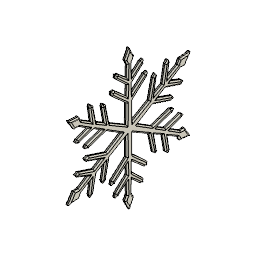
SnowFlake (Autodesk Fusion 360 design; units mm, degrees)
part number: 2026-06-10-18-37-35-509
Autodesk Fusion 360 part; units mm, degrees
sketch "Sketch1" plane through (0, 0, 0) normal (1, 0, 0) x (0, 1, 0)
  line L0 (-5.5093, 0.4362) -> (-18.2005, -7.4756)
  line L1 (-18.2005, -7.4756) -> (-32.6565, -2.7689)
  line L2 (-32.6565, -2.7689) -> (-35.5141, -3.6935)
  line L3 (-35.5141, -3.6935) -> (-34.2955, -5.7106)
  line L4 (-34.2955, -5.7106) -> (-22, -10)
  line L5 (-22, -10) -> (-28.4, -14)
  line L6 (-28.4, -14) -> (-40.4994, -10)
  line L7 (-40.4994, -10) -> (-42.867, -11.2872)
  line L8 (-42.867, -11.2872) -> (-41.5321, -12.9244)
  line L9 (-41.5321, -12.9244) -> (-32.5, -16.5)
  line L10 (-32.5, -16.5) -> (-40.363, -21.503)
  line L11 (-40.363, -21.503) -> (-44, -21.503)
  line L12 (-44, -21.503) -> (-48.7199, -28.8845)
  line L13 (-48.7199, -28.8845) -> (-40.1679, -28.1366)
  line L14 (-40.1679, -28.1366) -> (-38.477, -24.8523)
  line L15 (-38.477, -24.8523) -> (-30.5752, -19.9422)
  line L16 (-30.5752, -19.9422) -> (-32, -30)
  line L17 (-32, -30) -> (-31.2876, -32.0639)
  line L18 (-31.2876, -32.0639) -> (-28.76, -30)
  line L19 (-28.76, -30) -> (-26.2945, -17.4786)
  line L20 (-26.2945, -17.4786) -> (-19.6702, -13.6466)
  line L21 (-19.6702, -13.6466) -> (-21.809, -25.4099)
  line L22 (-21.809, -25.4099) -> (-21.0366, -27.3705)
  line L23 (-21.0366, -27.3705) -> (-18.779, -25.707)
  line L24 (-18.779, -25.707) -> (-15.8085, -11.5376)
  line L25 (-15.8085, -11.5376) -> (-2.5006, -3.7251)
  line L26 (-2.5006, -3.7251) -> (-2.2468, -18.655)
  line L27 (-2.2468, -18.655) -> (-14.0686, -29.3557)
  line L28 (-14.0686, -29.3557) -> (-14.5366, -32.1245)
  line L29 (-14.5366, -32.1245) -> (-11.9615, -32.0807)
  line L30 (-11.9615, -32.0807) -> (-2.2133, -23.506)
  line L31 (-2.2133, -23.506) -> (-1.8623, -31.1496)
  line L32 (-1.8623, -31.1496) -> (-10.9878, -39.6121)
  line L33 (-10.9878, -39.6121) -> (-11.3193, -42.4278)
  line L34 (-11.3193, -42.4278) -> (-9, -42)
  line L35 (-9, -42) -> (-2, -36)
  line L36 (-2, -36) -> (-1.7726, -45.2005)
  line L37 (-1.7726, -45.2005) -> (-3.5977, -48.4646)
  line L38 (-3.5977, -48.4646) -> (0.0525, -55.765)
  line L39 (0.0525, -55.765) -> (3.5974, -48.6752)
  line L40 (3.5974, -48.6752) -> (1.825, -45.1303)
  line L41 (1.825, -45.1303) -> (1.9829, -35.8293)
  line L42 (1.9829, -35.8293) -> (9, -42)
  line L43 (9, -42) -> (11.1435, -42.4628)
  line L44 (11.1435, -42.4628) -> (11.1906, -39.6913)
  line L45 (11.1906, -39.6913) -> (2, -31)
  line L46 (2, -31) -> (2.1281, -23.4568)
  line L47 (2.1281, -23.4568) -> (11.835, -31.9103)
  line L48 (11.835, -31.9103) -> (14.5094, -32.2339)
  line L49 (14.5094, -32.2339) -> (14.1643, -29.4085)
  line L50 (14.1643, -29.4085) -> (2.3645, -18.7108)
  line L51 (2.3645, -18.7108) -> (2.5306, -3.7879)
  line L52 (2.5306, -3.7879) -> (15.7927, -11.4272)
  line L53 (15.7927, -11.4272) -> (18.9089, -25.8047)
  line L54 (18.9089, -25.8047) -> (20.9993, -27.4018)
  line L55 (20.9993, -27.4018) -> (21.9193, -25.8047)
  line L56 (21.9193, -25.8047) -> (19.731, -13.7321)
  line L57 (19.731, -13.7321) -> (26.378, -17.3962)
  line L58 (26.378, -17.3962) -> (28.6992, -30.2019)
  line L59 (28.6992, -30.2019) -> (30.958, -32.1933)
  line L60 (30.958, -32.1933) -> (32.0558, -30.2019)
  line L61 (32.0558, -30.2019) -> (30.4413, -20.1912)
  line L62 (30.4413, -20.1912) -> (38.4975, -24.7712)
  line L63 (38.4975, -24.7712) -> (40, -28)
  line L64 (40, -28) -> (48.6207, -28.8816)
  line L65 (48.6207, -28.8816) -> (44.1111, -21.6239)
  line L66 (44.1111, -21.6239) -> (40.4, -21.6239)
  line L67 (40.4, -21.6239) -> (32.3908, -16.5271)
  line L68 (32.3908, -16.5271) -> (41.1281, -13.1449)
  line L69 (41.1281, -13.1449) -> (42.9367, -11.5947)
  line L70 (42.9367, -11.5947) -> (40.7993, -9.8802)
  line L71 (40.7993, -9.8802) -> (28.3998, -13.9874)
  line L72 (28.3998, -13.9874) -> (22, -10)
  line L73 (22, -10) -> (34.0584, -5.7229)
  line L74 (34.0584, -5.7229) -> (35.4207, -3.7499)
  line L75 (35.4207, -3.7499) -> (32.7431, -2.8104)
  line L76 (32.7431, -2.8104) -> (18.2936, -7.5314)
  line L77 (18.2936, -7.5314) -> (5.4788, 0.452)
  line L78 (5.4788, 0.452) -> (18.0611, 8.4612)
  line L79 (18.0611, 8.4612) -> (32.6327, 4.2758)
  line L80 (32.6327, 4.2758) -> (35.3972, 5.1542)
  line L81 (35.3972, 5.1542) -> (34.3896, 7.1436)
  line L82 (34.3896, 7.1436) -> (22.1432, 11.0707)
  line L83 (22.1432, 11.0707) -> (28.2664, 15.5662)
  line L84 (28.2664, 15.5662) -> (40.5644, 12.0525)
  line L85 (40.5644, 12.0525) -> (42.993, 13.4476)
  line L86 (42.993, 13.4476) -> (41.6496, 14.9978)
  line L87 (41.6496, 14.9978) -> (32.5552, 18.0207)
  line L88 (32.5552, 18.0207) -> (40.2802, 23.2654)
  line L89 (40.2802, 23.2654) -> (44, 23.2654)
  line L90 (44, 23.2654) -> (48.7804, 30.5254)
  line L91 (48.7804, 30.5254) -> (40.1252, 29.802)
  line L92 (40.1252, 29.802) -> (38.5492, 26.5466)
  line L93 (38.5492, 26.5466) -> (30.54, 21.5861)
  line L94 (30.54, 21.5861) -> (32.0643, 31.5847)
  line L95 (32.0643, 31.5847) -> (31.3021, 33.5741)
  line L96 (31.3021, 33.5741) -> (28.7056, 31.7397)
  line L97 (28.7056, 31.7397) -> (26.432, 19.0541)
  line L98 (26.432, 19.0541) -> (19.5854, 14.7911)
  line L99 (19.5854, 14.7911) -> (21.689, 26.5281)
  line L100 (21.689, 26.5281) -> (21.0581, 28.5877)
  line L101 (21.0581, 28.5877) -> (18.707, 26.9342)
  line L102 (18.707, 26.9342) -> (15.7616, 12.6726)
  line L103 (15.7616, 12.6726) -> (2.611, 4.7667)
  line L104 (2.611, 4.7667) -> (2.3009, 19.5967)
  line L105 (2.3009, 19.5967) -> (14.0978, 30.3084)
  line L106 (14.0978, 30.3084) -> (14.6093, 33.4346)
  line L107 (14.6093, 33.4346) -> (11.9379, 33.1504)
  line L108 (11.9379, 33.1504) -> (2.1046, 24.5107)
  line L109 (2.1046, 24.5107) -> (1.9384, 32.0866)
  line L110 (1.9384, 32.0866) -> (11, 41)
  line L111 (11, 41) -> (11.3126, 43.6942)
  line L112 (11.3126, 43.6942) -> (9.0005, 43.4482)
  line L113 (9.0005, 43.4482) -> (2, 37)
  line L114 (2, 37) -> (1.8204, 46.6783)
  line L115 (1.8204, 46.6783) -> (3.6677, 50.0034)
  line L116 (3.6677, 50.0034) -> (0.1152, 57.3073)
  line L117 (0.1152, 57.3073) -> (-3.7215, 50.0034)
  line L118 (-3.7215, 50.0034) -> (-1.8032, 46.6783)
  line L119 (-1.8032, 46.6783) -> (-1.9595, 37.1576)
  line L120 (-1.9595, 37.1576) -> (-8.8087, 43.2679)
  line L121 (-8.8087, 43.2679) -> (-11.1391, 43.7226)
  line L122 (-11.1391, 43.7226) -> (-11.1391, 41.108)
  line L123 (-11.1391, 41.108) -> (-2.0397, 32.2702)
  line L124 (-2.0397, 32.2702) -> (-2.0397, 24.5676)
  line L125 (-2.0397, 24.5676) -> (-11.8496, 33.2641)
  line L126 (-11.8496, 33.2641) -> (-14.4926, 33.463)
  line L127 (-14.4926, 33.463) -> (-14.1516, 30.4221)
  line L128 (-14.1516, 30.4221) -> (-2.3147, 19.6794)
  line L129 (-2.3147, 19.6794) -> (-2.5109, 4.8884)
  line L130 (-2.5109, 4.8884) -> (-15.6086, 12.2839)
  line L131 (-15.6086, 12.2839) -> (-18.6951, 26.8499)
  line L132 (-18.6951, 26.8499) -> (-20.7132, 28.7493)
  line L133 (-20.7132, 28.7493) -> (-21.7857, 26.8499)
  line L134 (-21.7857, 26.8499) -> (-19.7042, 14.9393)
  line L135 (-19.7042, 14.9393) -> (-26.4905, 18.8567)
  line L136 (-26.4905, 18.8567) -> (-28.7283, 31.6618)
  line L137 (-28.7283, 31.6618) -> (-30.9619, 33.6164)
  line L138 (-30.9619, 33.6164) -> (-31.9828, 31.8479)
  line L139 (-31.9828, 31.8479) -> (-30.5266, 21.5475)
  line L140 (-30.5266, 21.5475) -> (-38.322, 26.4938)
  line L141 (-38.322, 26.4938) -> (-40.0235, 29.5803)
  line L142 (-40.0235, 29.5803) -> (-48.6532, 30.3922)
  line L143 (-48.6532, 30.3922) -> (-44.192, 23.1657)
  line L144 (-44.192, 23.1657) -> (-40.2609, 23.2641)
  line L145 (-40.2609, 23.2641) -> (-32.5051, 18.184)
  line L146 (-32.5051, 18.184) -> (-41.4085, 15.0184)
  line L147 (-41.4085, 15.0184) -> (-42.8726, 13.4356)
  line L148 (-42.8726, 13.4356) -> (-40.5763, 11.9316)
  line L149 (-40.5763, 11.9316) -> (-28.5486, 15.5925)
  line L150 (-28.5486, 15.5925) -> (-21.9283, 11.2561)
  line L151 (-21.9283, 11.2561) -> (-34.2067, 7.1835)
  line L152 (-34.2067, 7.1835) -> (-35.4762, 5.2453)
  line L153 (-35.4762, 5.2453) -> (-32.703, 4.2949)
  line L154 (-32.703, 4.2949) -> (-18.2994, 8.5289)
  line L155 (-18.2994, 8.5289) -> (-5.5093, 0.4362)
  constraint horizontal L11
  constraint perpendicular L26 L29
  constraint parallel L38 L40
  constraint parallel L41 L44
  constraint parallel L44 L46
  constraint perpendicular L52 L55
  constraint parallel L56 L58
  constraint perpendicular L57 L60
  constraint horizontal L66
  constraint horizontal L89
  constraint parallel L97 L99
  constraint parallel L107 L112
  constraint vertical L122
  constraint parallel L122 L124
  constraint perpendicular L130 L133
  constraint parallel L134 L136
  constraint perpendicular L135 L138
  constraint parallel L145 L148
  constraint parallel L148 L150
  constraint perpendicular L150 L152
extrude "Extrude1" add sketch "Sketch1" along normal blind 1.5 makes body 1
fillet "Fillet1" radius 1 78 edges at (0, -11.8549, -3.5197) (0, -25.4285, -5.1223) (0, -34.0853, -3.2312) (0, -34.9048, -4.702) (0, -28.1477, -7.8553) (0, -25.2, -12) (0, -34.4497, -12) (0, -41.6832, -10.6436) (0, -42.1995, -12.1058) (0, -37.016, -14.7122) (0, -36.4315, -19.0015) (0, -42.1815, -21.503) (0, -46.36, -25.1937) (0, -44.4439, -28.5105) (0, -39.3224, -26.4944) (0, -34.5261, -22.3972) (0, -31.2876, -24.9711) (0, -31.6438, -31.0319) (0, -30.0238, -31.0319) (0, -27.5272, -23.7393) (0, -22.9823, -15.5626) (0, -20.7396, -19.5283) (0, -21.4228, -26.3902) (0, -19.9078, -26.5387) (0, -17.2938, -18.6223) (0, -9.1546, -7.6313) (0, -2.3737, -11.1901) (0, -8.1577, -24.0054) (0, -14.3026, -30.7401) (0, -13.249, -32.1026) (0, -7.0874, -27.7934) (0, -2.0378, -27.3278) (0, -6.425, -35.3808) (0, -11.1535, -41.0199) (0, -10.1596, -42.2139) (0, -5.5, -39) (0, -1.8863, -40.6003) (0, -2.6851, -46.8326) (0, -1.7726, -52.1148) (0, 1.825, -52.2201) (0, 2.7112, -46.9028) (0, 1.9039, -40.4798) (0, 5.4915, -38.9147) (0, 10.0718, -42.2314) (0, 11.167, -41.0771) (0, 6.5953, -35.3457) (0, 2.064, -27.2284) (0, 6.9815, -27.6836) (0, 13.1722, -32.0721) (0, 14.3369, -30.8212) (0, 8.2644, -24.0596) (0, 2.4475, -11.2493) (0, 9.1616, -7.6076) (0, 17.3508, -18.616) (0, 19.9541, -26.6033) (0, 21.4593, -26.6033) (0, 20.8252, -19.7684) (0, 23.0545, -15.5641) (0, 27.5386, -23.799) (0, 29.8286, -31.1976) (0, 31.5069, -31.1976) (0, 31.2486, -25.1965) (0, 34.4694, -22.4812) (0, 39.2488, -26.3856) (0, 44.3103, -28.4408) (0, 46.3659, -25.2527) (0, 42.2555, -21.6239) (0, 36.3954, -19.0755) (0, 36.7595, -14.836) (0, 42.0324, -12.3698) (0, 41.868, -10.7375) (0, 34.5996, -11.9338) (0, 25.1999, -11.9937) (0, 28.0292, -7.8614) (0, 34.7395, -4.7364) (0, 34.0819, -3.2802) (0, 25.5183, -5.1709) (0, 11.8862, -3.5397) on bodies 1
split "Split1" by plane through (0, 0, 0) normal (0, 0, 1) bodies 1 makes body 2 at (1.5, 44.3019, 27.8643)
delete_body "RemoveBody1" bodies 2
mirror "Mirror1" about plane through (0, 0, 0) normal (0, 0, 1) of bodies 1 merged
mirror "Mirror2" about plane through (1.5, 0, 0) normal (1, 0, 0) of bodies 1 merged
